Autodesk Fusion 360 part; units mm, degrees
(part 2 of 3)
  line L996 (25.447, -24.192) -> (26.789, -22.378)
  line L997 (26.789, -22.378) -> (26.864, -22.353)
  line L998 (25, -29.138) -> (25.075, -29.163)
  line L999 (25.075, -29.163) -> (26.118, -30.629)
  line L1000 (26.118, -30.629) -> (25.919, -31.026)
  line L1001 (25.919, -31.026) -> (25.025, -32.418)
  line L1002 (25.025, -32.418) -> (24.975, -32.418)
  line L1003 (24.975, -32.418) -> (24.826, -32.219)
  line L1004 (24.826, -32.219) -> (23.907, -30.703)
  line L1005 (23.907, -30.703) -> (23.907, -30.629)
  line L1006 (23.907, -30.629) -> (25, -29.138)
  line L1007 (25, -24.838) -> (25.05, -24.838)
  line L1008 (25.05, -24.838) -> (26.118, -26.354)
  line L1009 (26.118, -26.354) -> (26.118, -26.404)
  line L1010 (26.118, -26.404) -> (25.05, -27.87)
  line L1011 (25.05, -27.87) -> (24.975, -27.87)
  line L1012 (24.975, -27.87) -> (23.907, -26.404)
  line L1013 (23.907, -26.404) -> (23.907, -26.33)
  line L1014 (23.907, -26.33) -> (24.354, -25.683)
  line L1015 (24.354, -25.683) -> (25, -24.838)
  line L1016 (26.491, -27.025) -> (26.566, -27.025)
  line L1017 (26.566, -27.025) -> (26.64, -27.1)
  line L1018 (26.64, -27.1) -> (27.435, -28.268)
  line L1019 (27.435, -28.268) -> (27.435, -28.492)
  line L1020 (27.435, -28.492) -> (26.541, -29.983)
  line L1021 (26.541, -29.983) -> (26.466, -29.958)
  line L1022 (26.466, -29.958) -> (25.447, -28.566)
  line L1023 (25.447, -28.566) -> (25.447, -28.492)
  line L1024 (25.447, -28.492) -> (26.491, -27.025)
  line L1025 (23.459, -27) -> (23.534, -27.025)
  line L1026 (23.534, -27.025) -> (24.578, -28.492)
  line L1027 (24.578, -28.492) -> (24.478, -28.69)
  line L1028 (24.478, -28.69) -> (23.534, -29.983)
  line L1029 (23.534, -29.983) -> (23.484, -29.983)
  line L1030 (23.484, -29.983) -> (23.335, -29.784)
  line L1031 (23.335, -29.784) -> (22.589, -28.516)
  line L1032 (22.589, -28.516) -> (22.614, -28.243)
  line L1033 (22.614, -28.243) -> (23.459, -27)
  line L1034 (20.775, -19.346) -> (20.85, -19.371)
  line L1035 (20.85, -19.371) -> (21.421, -20.042)
  line L1036 (21.421, -20.042) -> (22.714, -21.682)
  line L1037 (22.714, -21.682) -> (22.714, -21.757)
  line L1038 (22.714, -21.757) -> (22.068, -22.975)
  line L1039 (22.068, -22.975) -> (21.993, -22.95)
  line L1040 (21.993, -22.95) -> (21.546, -21.409)
  line L1041 (21.546, -21.409) -> (20.999, -19.943)
  line L1042 (20.999, -19.943) -> (20.75, -19.421)
  line L1043 (20.75, -19.421) -> (20.775, -19.346)
  line L1044 (29.25, -19.346) -> (29.274, -19.421)
  line L1045 (29.274, -19.421) -> (28.951, -20.142)
  line L1046 (28.951, -20.142) -> (28.479, -21.434)
  line L1047 (28.479, -21.434) -> (28.057, -22.9)
  line L1048 (28.057, -22.9) -> (27.957, -22.95)
  line L1049 (27.957, -22.95) -> (27.56, -22.229)
  line L1050 (27.56, -22.229) -> (27.311, -21.682)
  line L1051 (27.311, -21.682) -> (28.28, -20.44)
  line L1052 (28.28, -20.44) -> (29.175, -19.371)
  line L1053 (29.175, -19.371) -> (29.25, -19.346)
  line L1054 (12.972, -15.072) -> (13.519, -15.047)
  line L1055 (13.519, -15.047) -> (13.917, -15.097)
  line L1056 (13.917, -15.097) -> (14.438, -15.221)
  line L1057 (14.438, -15.221) -> (15.383, -15.668)
  line L1058 (15.383, -15.668) -> (15.432, -15.768)
  line L1059 (15.432, -15.768) -> (15.333, -15.818)
  line L1060 (15.333, -15.818) -> (14.96, -15.867)
  line L1061 (14.96, -15.867) -> (14.563, -16.016)
  line L1062 (14.563, -16.016) -> (14.414, -16.016)
  line L1063 (14.414, -16.016) -> (13.593, -15.445)
  line L1064 (13.593, -15.445) -> (12.997, -15.147)
  line L1065 (12.997, -15.147) -> (12.972, -15.072)
  line L1066 (37.053, -15.072) -> (37.003, -15.171)
  line L1067 (37.003, -15.171) -> (36.804, -15.246)
  line L1068 (36.804, -15.246) -> (36.233, -15.569)
  line L1069 (36.233, -15.569) -> (35.611, -16.016)
  line L1070 (35.611, -16.016) -> (35.487, -16.016)
  line L1071 (35.487, -16.016) -> (35.338, -15.942)
  line L1072 (35.338, -15.942) -> (34.841, -15.818)
  line L1073 (34.841, -15.818) -> (34.692, -15.818)
  line L1074 (34.692, -15.818) -> (34.617, -15.768)
  line L1075 (34.617, -15.768) -> (34.667, -15.668)
  line L1076 (34.667, -15.668) -> (34.916, -15.519)
  line L1077 (34.916, -15.519) -> (35.76, -15.171)
  line L1078 (35.76, -15.171) -> (36.506, -15.047)
  line L1079 (36.506, -15.047) -> (37.053, -15.072)
  line L1080 (24.205, -7.517) -> (24.975, -7.12)
  line L1081 (24.975, -7.12) -> (25.075, -7.12)
  line L1082 (25.075, -7.12) -> (25.845, -7.493)
  line L1083 (25.845, -7.493) -> (25.87, -7.567)
  line L1084 (25.87, -7.567) -> (25, -7.99)
  line L1085 (25, -7.99) -> (24.254, -7.617)
  line L1086 (24.254, -7.617) -> (24.205, -7.517)
  line L1087 (27.46, -29.784) -> (27.535, -29.809)
  line L1088 (27.535, -29.809) -> (27.659, -30.877)
  line L1089 (27.659, -30.877) -> (27.808, -31.623)
  line L1090 (27.808, -31.623) -> (27.783, -31.747)
  line L1091 (27.783, -31.747) -> (27.709, -31.722)
  line L1092 (27.709, -31.722) -> (26.963, -30.654)
  line L1093 (26.963, -30.654) -> (26.988, -30.529)
  line L1094 (26.988, -30.529) -> (27.46, -29.784)
  line L1095 (22.565, -29.784) -> (23.037, -30.554)
  line L1096 (23.037, -30.554) -> (23.062, -30.654)
  line L1097 (23.062, -30.654) -> (22.341, -31.672)
  line L1098 (22.341, -31.672) -> (22.266, -31.697)
  line L1099 (22.266, -31.697) -> (22.242, -31.573)
  line L1100 (22.242, -31.573) -> (22.391, -30.753)
  line L1101 (22.391, -30.753) -> (22.49, -29.809)
  line L1102 (22.49, -29.809) -> (22.565, -29.784)
  line L1103 (27.535, -25.634) -> (27.56, -25.808)
  line L1104 (27.56, -25.808) -> (27.46, -26.951)
  line L1105 (27.46, -26.951) -> (27.386, -26.976)
  line L1106 (27.386, -26.976) -> (27.013, -26.479)
  line L1107 (27.013, -26.479) -> (26.988, -26.33)
  line L1108 (26.988, -26.33) -> (27.46, -25.659)
  line L1109 (27.46, -25.659) -> (27.535, -25.634)
  line L1110 (22.49, -25.634) -> (22.565, -25.659)
  line L1111 (22.565, -25.659) -> (23.037, -26.33)
  line L1112 (23.037, -26.33) -> (23.037, -26.429)
  line L1113 (23.037, -26.429) -> (22.639, -26.976)
  line L1114 (22.639, -26.976) -> (22.565, -26.951)
  line L1115 (22.565, -26.951) -> (22.565, -26.553)
  line L1116 (22.565, -26.553) -> (22.465, -25.708)
  line L1117 (22.465, -25.708) -> (22.49, -25.634)
extrude "Extrude1" add sketch "Sketch1" along normal blind 3
sketch "Sketch2" plane through (0, 0, 0) normal (0, 0, 1) x (1, 0, 0)
  circle A0 centre (25, -25) radius 27.5
  circle A1 centre (25, -25) radius 24
  line L0 (24.5, -0.5) -> (25.5, -0.5)
  line L1 (25.5, -0.5) -> (25.5, -6.5)
  line L2 (25.5, -6.5) -> (24.5, -6.5)
  line L3 (24.5, -6.5) -> (24.5, -0.5)
  line L4 (11.009, -44.421) -> (19.21, -44.396)
  line L5 (13.345, -43.725) -> (12.202, -43.7)
  line L6 (37.823, -43.7) -> (36.705, -43.725)
  line L7 (30.691, -44.396) -> (39.041, -44.396)
  line L8 (37.264, -43.7125) -> (40.3407, -43.7125)
  line L9 (40.3407, -43.7125) -> (40.3407, -44.396)
  line L10 (40.3407, -44.396) -> (37.264, -44.396)
  line L11 (37.264, -44.396) -> (37.264, -43.7125)
  line L12 (12.7735, -43.7125) -> (9.7904, -43.7125)
  line L13 (9.7904, -43.7125) -> (9.7904, -44.4085)
  line L14 (9.7904, -44.4085) -> (12.7735, -44.4085)
  line L15 (12.7735, -44.4085) -> (12.7735, -43.7125)
  line L16 (12.351, -11.643) -> (7.306, -13.73)
  line L17 (7.654, -14.476) -> (14.612, -11.593)
  line L18 (42.719, -13.705) -> (39.19, -12.239)
  line L19 (38.917, -13.009) -> (42.371, -14.476)
  line L20 (40.9545, -12.972) -> (40.644, -13.7425)
  line L21 (40.644, -13.7425) -> (47.8102, -16.6302)
  line L22 (47.8102, -16.6302) -> (48.1207, -15.8597)
  line L23 (48.1207, -15.8597) -> (40.9545, -12.972)
  line L24 (9.8285, -12.6865) -> (10.1427, -13.4448)
  line L25 (10.1427, -13.4448) -> (2.127, -16.766)
  line L26 (2.127, -16.766) -> (1.8128, -16.0077)
  line L27 (1.8128, -16.0077) -> (9.8285, -12.6865)
  dimension "d3" = 55
  dimension "d4" = 48
  constraint concentric A0 A1
  constraint horizontal L0
  constraint vertical L1
  constraint horizontal L2
  constraint vertical L3
  constraint horizontal L8
  constraint vertical L9
  constraint horizontal L10
  constraint vertical L11
  constraint midpoint L6 L8.start
  constraint horizontal L12
  constraint vertical L13
  constraint horizontal L14
  constraint vertical L15
  constraint midpoint L5 L12.start
  constraint perpendicular L20 L21
  constraint parallel L20 L22
  constraint parallel L21 L23
  constraint midpoint L19 L20.end
  constraint midpoint L18 L20.start
  constraint perpendicular L24 L25
  constraint parallel L24 L26
  constraint parallel L25 L27
  constraint coincident L17 L24.end
  constraint perpendicular L17 L24
  constraint midpoint L16 L24.start
  measures "d3" diameter of A0
  measures "d4" diameter of A1
extrude "Extrude2" add sketch "Sketch2" along normal blind 3 contours A0 | A1 L20 L21 L23 | A1 L21 L22 L23 | A1 L8 L9 L10 | A1 L7 L8 L10 L11 | A1 L1 L2 L3 | A1 L0 L1 L3 | A1 L12 L13 L14 | A1 L12 L14 L15 | A1 L16 L17 L24 L25 L27 | A1 L25 L26 L27
sketch "Sketch4" plane through (0, 0, 3) normal (0, 0, 1) x (-1, 0, 0)
  arc A0 (-6.803, 9.3517) -> (-2.9434, 15.5393) centre (-25, 25) ccw
  line L0 (-11.1263, 43.7125) -> (-9.9976, 43.7125)
  line L1 (-24.5, 1.0052) -> (-24.5, 5.9525)
  line L2 (-25.5, 5.9758) -> (-25.5, 1.0052)
  line L3 (-40.0281, 43.7125) -> (-38.8766, 43.7125)
  line L4 (-30.691, 44.396) -> (-39.041, 44.396)
  circle A1 centre (-25, 25) radius 27.5
  circle A2 centre (-25, 25) radius 27.5
  circle A3 centre (-25, 25) radius 27.5
  circle A4 centre (-25, 25) radius 25.5
  line L5 (-24.5, 5.9525) -> (-22.639, 4.983)
  line L6 (-22.639, 4.983) -> (-21.993, 4.684)
  line L7 (-21.993, 4.684) -> (-21.645, 5.355)
  line L8 (-21.645, 5.355) -> (-21.695, 5.455)
  line L9 (-21.695, 5.455) -> (-24.006, 6.623)
  line L10 (-24.006, 6.623) -> (-23.981, 6.722)
  line L11 (-23.981, 6.722) -> (-23.236, 7.095)
  line L12 (-23.236, 7.095) -> (-22.913, 6.971)
  line L13 (-22.913, 6.971) -> (-19.135, 5.082)
  line L14 (-19.135, 5.082) -> (-19.036, 5.082)
  line L15 (-19.036, 5.082) -> (-18.738, 5.678)
  line L16 (-18.738, 5.678) -> (-18.713, 5.803)
  line L17 (-18.713, 5.803) -> (-18.762, 5.852)
  line L18 (-18.762, 5.852) -> (-22.142, 7.468)
  line L19 (-22.142, 7.468) -> (-22.167, 7.567)
  line L20 (-22.167, 7.567) -> (-18.588, 9.133)
  line L21 (-18.588, 9.133) -> (-12.351, 11.643)
  line L22 (-12.351, 11.643) -> (-7.306, 13.73)
  line L23 (-7.306, 13.73) -> (-7.3062, 13.7316)
  line L24 (-2.5162, 16.6048) -> (-14.612, 11.593)
  line L25 (-14.612, 11.593) -> (-14.687, 11.593)
  line L26 (-14.687, 11.593) -> (-14.786, 11.692)
  line L27 (-14.786, 11.692) -> (-15.234, 12.338)
  line L28 (-15.234, 12.338) -> (-15.283, 12.363)
  line L29 (-15.283, 12.363) -> (-15.283, 12.413)
  line L30 (-15.283, 12.413) -> (-15.184, 12.488)
  line L31 (-15.184, 12.488) -> (-11.257, 14.327)
  line L32 (-11.257, 14.327) -> (-10.736, 14.401)
  line L33 (-10.736, 14.401) -> (-9.568, 14.476)
  line L34 (-9.568, 14.476) -> (-8.822, 14.6)
  line L35 (-8.822, 14.6) -> (-7.878, 14.873)
  line L36 (-7.878, 14.873) -> (-6.909, 15.321)
  line L37 (-6.909, 15.321) -> (-6.064, 15.867)
  line L38 (-6.064, 15.867) -> (-5.442, 16.389)
  line L39 (-5.442, 16.389) -> (-4.722, 17.16)
  line L40 (-4.722, 17.16) -> (-4.125, 18.004)
  line L41 (-4.125, 18.004) -> (-3.628, 18.949)
  line L42 (-3.628, 18.949) -> (-3.28, 19.794)
  line L43 (-3.28, 19.794) -> (-2.908, 21.061)
  line L44 (-2.908, 21.061) -> (-2.709, 22.229)
  line L45 (-2.709, 22.229) -> (-2.609, 23.397)
  line L46 (-2.609, 23.397) -> (-2.609, 26.18)
  line L47 (-2.609, 26.18) -> (-2.46, 26.255)
  line L48 (-2.46, 26.255) -> (-2.386, 26.379)
  line L49 (-2.386, 26.379) -> (-2.411, 31.772)
  line L50 (-2.411, 31.772) -> (-2.56, 31.871)
  line L51 (-2.56, 31.871) -> (-3.429, 31.846)
  line L52 (-3.429, 31.846) -> (-3.529, 31.747)
  line L53 (-3.529, 31.747) -> (-3.529, 26.354)
  line L54 (-3.529, 26.354) -> (-3.454, 26.255)
  line L55 (-3.454, 26.255) -> (-3.305, 26.18)
  line L56 (-3.305, 26.18) -> (-3.33, 23.298)
  line L57 (-3.33, 23.298) -> (-3.405, 22.403)
  line L58 (-3.405, 22.403) -> (-3.529, 21.608)
  line L59 (-3.529, 21.608) -> (-3.802, 20.539)
  line L60 (-3.802, 20.539) -> (-4.15, 19.57)
  line L61 (-4.15, 19.57) -> (-4.548, 18.75)
  line L62 (-4.548, 18.75) -> (-5.119, 17.855)
  line L63 (-5.119, 17.855) -> (-5.567, 17.309)
  line L64 (-5.567, 17.309) -> (-6.362, 16.563)
  line L65 (-6.362, 16.563) -> (-7.083, 16.066)
  line L66 (-7.083, 16.066) -> (-7.853, 15.668)
  line L67 (-7.853, 15.668) -> (-8.549, 15.42)
  line L68 (-8.549, 15.42) -> (-9.493, 15.221)
  line L69 (-9.493, 15.221) -> (-10.437, 15.196)
  line L70 (-10.437, 15.196) -> (-10.487, 15.296)
  line L71 (-10.487, 15.296) -> (-9.965, 15.619)
  line L72 (-9.965, 15.619) -> (-9.195, 16.215)
  line L73 (-9.195, 16.215) -> (-8.499, 16.911)
  line L74 (-8.499, 16.911) -> (-7.977, 17.582)
  line L75 (-7.977, 17.582) -> (-7.455, 18.427)
  line L76 (-7.455, 18.427) -> (-7.083, 19.197)
  line L77 (-7.083, 19.197) -> (-6.759, 20.067)
  line L78 (-6.759, 20.067) -> (-6.436, 21.334)
  line L79 (-6.436, 21.334) -> (-6.312, 22.105)
  line L80 (-6.312, 22.105) -> (-6.213, 23.173)
  line L81 (-6.213, 23.173) -> (-6.213, 28.019)
  line L82 (-6.213, 28.019) -> (-6.188, 28.119)
  line L83 (-6.188, 28.119) -> (-6.039, 28.268)
  line L84 (-6.039, 28.268) -> (-6.039, 34.307)
  line L85 (-6.039, 34.307) -> (-6.163, 34.406)
  line L86 (-6.163, 34.406) -> (-7.058, 34.406)
  line L87 (-7.058, 34.406) -> (-7.182, 34.282)
  line L88 (-7.182, 34.282) -> (-7.182, 28.268)
  line L89 (-7.182, 28.268) -> (-7.058, 28.144)
  line L90 (-7.058, 28.144) -> (-6.958, 28.144)
  line L91 (-6.958, 28.144) -> (-6.909, 28.094)
  line L92 (-6.909, 28.094) -> (-6.909, 23.571)
  line L93 (-6.909, 23.571) -> (-6.983, 22.478)
  line L94 (-6.983, 22.478) -> (-7.058, 21.956)
  line L95 (-7.058, 21.956) -> (-7.381, 20.514)
  line L96 (-7.381, 20.514) -> (-7.629, 19.794)
  line L97 (-7.629, 19.794) -> (-8.077, 18.825)
  line L98 (-8.077, 18.825) -> (-8.499, 18.129)
  line L99 (-8.499, 18.129) -> (-9.046, 17.408)
  line L100 (-9.046, 17.408) -> (-9.717, 16.737)
  line L101 (-9.717, 16.737) -> (-10.288, 16.29)
  line L102 (-10.288, 16.29) -> (-11.108, 15.793)
  line L103 (-11.108, 15.793) -> (-11.655, 15.544)
  line L104 (-11.655, 15.544) -> (-11.953, 15.495)
  line L105 (-11.953, 15.495) -> (-12.525, 15.718)
  line L106 (-12.525, 15.718) -> (-13.37, 16.166)
  line L107 (-13.37, 16.166) -> (-13.593, 16.315)
  line L108 (-13.593, 16.315) -> (-13.643, 16.414)
  line L109 (-13.643, 16.414) -> (-13.121, 16.787)
  line L110 (-13.121, 16.787) -> (-12.724, 17.16)
  line L111 (-12.724, 17.16) -> (-12.401, 17.532)
  line L112 (-12.401, 17.532) -> (-11.978, 18.154)
  line L113 (-11.978, 18.154) -> (-11.754, 18.551)
  line L114 (-11.754, 18.551) -> (-11.307, 19.595)
  line L115 (-11.307, 19.595) -> (-11.059, 20.415)
  line L116 (-11.059, 20.415) -> (-10.91, 21.061)
  line L117 (-10.91, 21.061) -> (-10.785, 21.807)
  line L118 (-10.785, 21.807) -> (-10.661, 23.248)
  line L119 (-10.661, 23.248) -> (-10.686, 26.379)
  line L120 (-10.686, 26.379) -> (-10.661, 26.653)
  line L121 (-10.661, 26.653) -> (-10.562, 26.702)
  line L122 (-10.562, 26.702) -> (-10.462, 26.827)
  line L123 (-10.462, 26.827) -> (-10.487, 33.064)
  line L124 (-10.487, 33.064) -> (-10.586, 33.139)
  line L125 (-10.586, 33.139) -> (-11.506, 33.139)
  line L126 (-11.506, 33.139) -> (-11.605, 33.064)
  line L127 (-11.605, 33.064) -> (-11.63, 32.99)
  line L128 (-11.63, 32.99) -> (-11.63, 26.827)
  line L129 (-11.63, 26.827) -> (-11.531, 26.702)
  line L130 (-11.531, 26.702) -> (-11.407, 26.677)
  line L131 (-11.407, 26.677) -> (-11.357, 26.628)
  line L132 (-11.357, 26.628) -> (-11.357, 23.646)
  line L133 (-11.357, 23.646) -> (-11.481, 22.03)
  line L134 (-11.481, 22.03) -> (-11.655, 21.036)
  line L135 (-11.655, 21.036) -> (-12.003, 19.794)
  line L136 (-12.003, 19.794) -> (-12.251, 19.197)
  line L137 (-12.251, 19.197) -> (-12.649, 18.452)
  line L138 (-12.649, 18.452) -> (-13.022, 17.93)
  line L139 (-13.022, 17.93) -> (-13.469, 17.458)
  line L140 (-13.469, 17.458) -> (-13.743, 17.234)
  line L141 (-13.743, 17.234) -> (-14.314, 16.886)
  line L142 (-14.314, 16.886) -> (-14.364, 16.886)
  line L143 (-14.364, 16.886) -> (-15.283, 17.806)
  line L144 (-15.283, 17.806) -> (-15.656, 18.253)
  line L145 (-15.656, 18.253) -> (-16.352, 19.222)
  line L146 (-16.352, 19.222) -> (-16.923, 20.167)
  line L147 (-16.923, 20.167) -> (-17.321, 20.937)
  line L148 (-17.321, 20.937) -> (-18.017, 22.577)
  line L149 (-18.017, 22.577) -> (-18.489, 24.043)
  line L150 (-18.489, 24.043) -> (-18.688, 24.838)
  line L151 (-18.688, 24.838) -> (-18.887, 25.932)
  line L152 (-18.887, 25.932) -> (-19.036, 27.547)
  line L153 (-19.036, 27.547) -> (-19.011, 29.386)
  line L154 (-19.011, 29.386) -> (-18.812, 30.877)
  line L155 (-18.812, 30.877) -> (-18.415, 32.468)
  line L156 (-18.415, 32.468) -> (-18.216, 33.064)
  line L157 (-18.216, 33.064) -> (-17.52, 34.704)
  line L158 (-17.52, 34.704) -> (-16.874, 35.922)
  line L159 (-16.874, 35.922) -> (-15.979, 37.413)
  line L160 (-15.979, 37.413) -> (-14.314, 39.824)
  line L161 (-14.314, 39.824) -> (-12.798, 41.762)
  line L162 (-12.798, 41.762) -> (-11.1263, 43.7125)
  line L163 (-9.9976, 43.7125) -> (-9.568, 43.377)
  line L164 (-9.568, 43.377) -> (-8.8988, 42.7975)
  line L165 (-8.7235, 42.6374) -> (-8.2028, 42.1422)
  arc A5 (-2.5162, 16.6048) -> (-8.2028, 42.1422) centre (-25, 25) ccw
  line L166 (-6.803, 9.3517) -> (-6.9294, 9.2059)
  arc A6 (-7.6077, 8.4619) -> (-6.9294, 9.2059) centre (-25, 25) ccw
  line L167 (-7.6077, 8.4619) -> (-8.7441, 7.3437)
  arc A7 (-24.5, 1.0052) -> (-8.7441, 7.3437) centre (-25, 25) ccw
  line L168 (-37.823, 43.7) -> (-36.705, 43.725)
  line L169 (-36.705, 43.725) -> (-36.605, 43.675)
  line L170 (-36.605, 43.675) -> (-34.742, 41.315)
  line L171 (-34.742, 41.315) -> (-33.772, 39.948)
  line L172 (-33.772, 39.948) -> (-32.753, 38.382)
  line L173 (-32.753, 38.382) -> (-32.107, 37.264)
  line L174 (-32.107, 37.264) -> (-31.561, 36.195)
  line L175 (-31.561, 36.195) -> (-30.865, 34.555)
  line L176 (-30.865, 34.555) -> (-30.467, 33.412)
  line L177 (-30.467, 33.412) -> (-30.219, 32.542)
  line L178 (-30.219, 32.542) -> (-29.995, 31.598)
  line L179 (-29.995, 31.598) -> (-29.821, 30.629)
  line L180 (-29.821, 30.629) -> (-29.647, 29.138)
  line L181 (-29.647, 29.138) -> (-29.622, 27.274)
  line L182 (-29.622, 27.274) -> (-29.821, 25.261)
  line L183 (-29.821, 25.261) -> (-30.244, 23.298)
  line L184 (-30.244, 23.298) -> (-30.517, 22.378)
  line L185 (-30.517, 22.378) -> (-30.989, 21.061)
  line L186 (-30.989, 21.061) -> (-31.809, 19.247)
  line L187 (-31.809, 19.247) -> (-32.306, 18.352)
  line L188 (-32.306, 18.352) -> (-32.828, 17.532)
  line L189 (-32.828, 17.532) -> (-33.648, 16.513)
  line L190 (-33.648, 16.513) -> (-34.468, 16.513)
  line L191 (-34.468, 16.513) -> (-34.816, 16.588)
  line L192 (-34.816, 16.588) -> (-34.841, 16.663)
  line L193 (-34.841, 16.663) -> (-34.319, 17.184)
  line L194 (-34.319, 17.184) -> (-33.623, 18.029)
  line L195 (-33.623, 18.029) -> (-33.101, 18.775)
  line L196 (-33.101, 18.775) -> (-32.455, 19.843)
  line L197 (-32.455, 19.843) -> (-31.635, 21.558)
  line L198 (-31.635, 21.558) -> (-30.989, 23.372)
  line L199 (-30.989, 23.372) -> (-30.741, 24.292)
  line L200 (-30.741, 24.292) -> (-30.542, 25.236)
  line L201 (-30.542, 25.236) -> (-30.293, 27.174)
  line L202 (-30.293, 27.174) -> (-30.268, 28.765)
  line L203 (-30.268, 28.765) -> (-30.417, 30.38)
  line L204 (-30.417, 30.38) -> (-30.741, 31.971)
  line L205 (-30.741, 31.971) -> (-31.188, 33.412)
  line L206 (-31.188, 33.412) -> (-31.71, 34.679)
  line L207 (-31.71, 34.679) -> (-32.455, 36.146)
  line L208 (-32.455, 36.146) -> (-33.499, 37.885)
  line L209 (-33.499, 37.885) -> (-34.766, 39.749)
  line L210 (-34.766, 39.749) -> (-36.357, 41.861)
  line L211 (-36.357, 41.861) -> (-37.848, 43.626)
  line L212 (-37.848, 43.626) -> (-37.823, 43.7)
  line L213 (-21.421, 34.878) -> (-21.595, 34.232)
  line L214 (-21.595, 34.232) -> (-21.67, 34.207)
  line L215 (-21.67, 34.207) -> (-21.769, 34.406)
  line L216 (-21.769, 34.406) -> (-22.291, 35.997)
  line L217 (-22.291, 35.997) -> (-22.465, 36.419)
  line L218 (-22.465, 36.419) -> (-22.515, 36.667)
  line L219 (-22.515, 36.667) -> (-20.8, 39.55)
  line L220 (-20.8, 39.55) -> (-19.98, 41.016)
  line L221 (-19.98, 41.016) -> (-19.185, 42.607)
  line L222 (-19.185, 42.607) -> (-18.762, 43.675)
  line L223 (-18.762, 43.675) -> (-18.688, 43.725)
  line L224 (-18.688, 43.725) -> (-17.768, 43.725)
  line L225 (-17.768, 43.725) -> (-17.719, 43.675)
  line L226 (-17.719, 43.675) -> (-17.744, 43.551)
  line L227 (-17.744, 43.551) -> (-18.986, 41.016)
  line L228 (-18.986, 41.016) -> (-20.179, 38.258)
  line L229 (-20.179, 38.258) -> (-20.949, 36.27)
  line L230 (-20.949, 36.27) -> (-21.421, 34.878)
  line L231 (-30.915, 17.756) -> (-31.436, 16.911)
  line L232 (-31.436, 16.911) -> (-31.735, 16.513)
  line L233 (-31.735, 16.513) -> (-32.604, 16.513)
  line L234 (-32.604, 16.513) -> (-32.629, 16.588)
  line L235 (-32.629, 16.588) -> (-32.281, 17.035)
  line L236 (-32.281, 17.035) -> (-31.561, 18.178)
  line L237 (-31.561, 18.178) -> (-30.815, 19.62)
  line L238 (-30.815, 19.62) -> (-30.442, 20.465)
  line L239 (-30.442, 20.465) -> (-30.094, 21.359)
  line L240 (-30.094, 21.359) -> (-29.722, 22.478)
  line L241 (-29.722, 22.478) -> (-29.25, 24.366)
  line L242 (-29.25, 24.366) -> (-29.001, 25.957)
  line L243 (-29.001, 25.957) -> (-28.902, 27.398)
  line L244 (-28.902, 27.398) -> (-28.926, 29.138)
  line L245 (-28.926, 29.138) -> (-29.051, 30.331)
  line L246 (-29.051, 30.331) -> (-29.349, 31.971)
  line L247 (-29.349, 31.971) -> (-29.771, 33.586)
  line L248 (-29.771, 33.586) -> (-29.97, 34.207)
  line L249 (-29.97, 34.207) -> (-30.492, 35.549)
  line L250 (-30.492, 35.549) -> (-31.064, 36.792)
  line L251 (-31.064, 36.792) -> (-31.759, 38.109)
  line L252 (-31.759, 38.109) -> (-32.654, 39.575)
  line L253 (-32.654, 39.575) -> (-33.971, 41.489)
  line L254 (-33.971, 41.489) -> (-35.487, 43.452)
  line L255 (-35.487, 43.452) -> (-35.661, 43.626)
  line L256 (-35.661, 43.626) -> (-35.636, 43.725)
  line L257 (-35.636, 43.725) -> (-33.077, 43.725)
  line L258 (-33.077, 43.725) -> (-33.002, 43.675)
  line L259 (-33.002, 43.675) -> (-31.809, 41.091)
  line L260 (-31.809, 41.091) -> (-31.784, 40.967)
  line L261 (-31.784, 40.967) -> (-31.735, 40.917)
  line L262 (-31.735, 40.917) -> (-30.268, 37.363)
  line L263 (-30.268, 37.363) -> (-29.573, 35.475)
  line L264 (-29.573, 35.475) -> (-28.926, 33.412)
  line L265 (-28.926, 33.412) -> (-28.628, 32.169)
  line L266 (-28.628, 32.169) -> (-28.33, 30.554)
  line L267 (-28.33, 30.554) -> (-28.181, 29.138)
  line L268 (-28.181, 29.138) -> (-28.156, 27.224)
  line L269 (-28.156, 27.224) -> (-28.33, 25.186)
  line L270 (-28.33, 25.186) -> (-28.653, 23.472)
  line L271 (-28.653, 23.472) -> (-28.951, 22.329)
  line L272 (-28.951, 22.329) -> (-29.25, 21.434)
  line L273 (-29.25, 21.434) -> (-29.92, 19.719)
  line L274 (-29.92, 19.719) -> (-30.517, 18.477)
  line L275 (-30.517, 18.477) -> (-30.915, 17.756)
  line L276 (-22.465, 10.077) -> (-23.111, 9.829)
  line L277 (-23.111, 9.829) -> (-24.975, 8.909)
  line L278 (-24.975, 8.909) -> (-25.075, 8.909)
  line L279 (-25.075, 8.909) -> (-26.789, 9.754)
  line L280 (-26.789, 9.754) -> (-27.584, 10.077)
  line L281 (-27.584, 10.077) -> (-27.709, 10.226)
  line L282 (-27.709, 10.226) -> (-28.355, 11.295)
  line L283 (-28.355, 11.295) -> (-28.305, 11.469)
  line L284 (-28.305, 11.469) -> (-26.69, 14.202)
  line L285 (-26.69, 14.202) -> (-25.919, 15.594)
  line L286 (-25.919, 15.594) -> (-25.845, 15.668)
  line L287 (-25.845, 15.668) -> (-25.447, 15.668)
  line L288 (-25.447, 15.668) -> (-25.398, 15.619)
  line L289 (-25.398, 15.619) -> (-25.398, 13.879)
  line L290 (-25.398, 13.879) -> (-25.348, 13.854)
  line L291 (-25.348, 13.854) -> (-24.677, 13.854)
  line L292 (-24.677, 13.854) -> (-24.627, 13.904)
  line L293 (-24.627, 13.904) -> (-24.627, 15.619)
  line L294 (-24.627, 15.619) -> (-24.578, 15.668)
  line L295 (-24.578, 15.668) -> (-24.205, 15.668)
  line L296 (-24.205, 15.668) -> (-24.105, 15.569)
  line L297 (-24.105, 15.569) -> (-21.67, 11.369)
  line L298 (-21.67, 11.369) -> (-21.67, 11.295)
  line L299 (-21.67, 11.295) -> (-22.266, 10.326)
  line L300 (-22.266, 10.326) -> (-22.465, 10.077)
  line L301 (-34.195, 13.109) -> (-34.418, 13.159)
  line L302 (-34.418, 13.159) -> (-36.73, 14.252)
  line L303 (-36.73, 14.252) -> (-36.705, 14.327)
  line L304 (-36.705, 14.327) -> (-36.108, 14.351)
  line L305 (-36.108, 14.351) -> (-35.537, 14.476)
  line L306 (-35.537, 14.476) -> (-34.866, 14.724)
  line L307 (-34.866, 14.724) -> (-34.195, 15.097)
  line L308 (-34.195, 15.097) -> (-33.474, 15.668)
  line L309 (-33.474, 15.668) -> (-32.406, 15.644)
  line L310 (-32.406, 15.644) -> (-32.43, 15.544)
  line L311 (-32.43, 15.544) -> (-34.195, 13.109)
  line L312 (-18.216, 11.941) -> (-21.098, 10.649)
  line L313 (-21.098, 10.649) -> (-21.173, 10.649)
  line L314 (-21.173, 10.649) -> (-21.198, 10.748)
  line L315 (-21.198, 10.748) -> (-18.588, 15.072)
  line L316 (-18.588, 15.072) -> (-18.464, 15.271)
  line L317 (-18.464, 15.271) -> (-18.365, 15.321)
  line L318 (-18.365, 15.321) -> (-16.526, 12.811)
  line L319 (-16.526, 12.811) -> (-16.526, 12.761)
  line L320 (-16.526, 12.761) -> (-16.998, 12.512)
  line L321 (-16.998, 12.512) -> (-18.017, 12.065)
  line L322 (-18.017, 12.065) -> (-18.216, 11.941)
  line L323 (-13.693, 14.327) -> (-13.345, 14.327)
  line L324 (-13.345, 14.327) -> (-13.32, 14.252)
  line L325 (-13.32, 14.252) -> (-15.731, 13.109)
  line L326 (-15.731, 13.109) -> (-15.83, 13.109)
  line L327 (-15.83, 13.109) -> (-17.644, 15.594)
  line L328 (-17.644, 15.594) -> (-17.644, 15.644)
  line L329 (-17.644, 15.644) -> (-16.551, 15.668)
  line L330 (-16.551, 15.668) -> (-16.153, 15.321)
  line L331 (-16.153, 15.321) -> (-15.606, 14.948)
  line L332 (-15.606, 14.948) -> (-15.01, 14.65)
  line L333 (-15.01, 14.65) -> (-14.314, 14.426)
  line L334 (-14.314, 14.426) -> (-13.693, 14.327)
  line L335 (-23.907, 30.703) -> (-23.907, 30.629)
  line L336 (-23.907, 30.629) -> (-25, 29.138)
  line L337 (-25, 29.138) -> (-25.075, 29.163)
  line L338 (-25.075, 29.163) -> (-26.118, 30.629)
  line L339 (-26.118, 30.629) -> (-25.919, 31.026)
  line L340 (-25.919, 31.026) -> (-25.025, 32.418)
  line L341 (-25.025, 32.418) -> (-24.975, 32.418)
  line L342 (-24.975, 32.418) -> (-24.826, 32.219)
  line L343 (-24.826, 32.219) -> (-23.907, 30.703)
  line L344 (-26.963, 30.654) -> (-26.988, 30.529)
  line L345 (-26.988, 30.529) -> (-27.46, 29.784)
  line L346 (-27.46, 29.784) -> (-27.535, 29.809)
  line L347 (-27.535, 29.809) -> (-27.659, 30.877)
  line L348 (-27.659, 30.877) -> (-27.808, 31.623)
  line L349 (-27.808, 31.623) -> (-27.783, 31.747)
  line L350 (-27.783, 31.747) -> (-27.709, 31.722)
  line L351 (-27.709, 31.722) -> (-26.963, 30.654)
  line L352 (-25, 7.99) -> (-24.254, 7.617)
  line L353 (-24.254, 7.617) -> (-24.205, 7.517)
  line L354 (-24.205, 7.517) -> (-24.975, 7.12)
  line L355 (-24.975, 7.12) -> (-25.075, 7.12)
  line L356 (-25.075, 7.12) -> (-25.845, 7.493)
  line L357 (-25.845, 7.493) -> (-25.87, 7.567)
  line L358 (-25.87, 7.567) -> (-25, 7.99)
  line L359 (-29.15, 11.245) -> (-28.802, 10.698)
  line L360 (-28.802, 10.698) -> (-28.827, 10.624)
  line L361 (-28.827, 10.624) -> (-30.144, 11.17)
  line L362 (-30.144, 11.17) -> (-33.499, 12.736)
  line L363 (-33.499, 12.736) -> (-33.499, 12.811)
  line L364 (-33.499, 12.811) -> (-32.207, 14.55)
  line L365 (-32.207, 14.55) -> (-31.66, 15.345)
  line L366 (-31.66, 15.345) -> (-31.561, 15.296)
  line L367 (-31.561, 15.296) -> (-31.412, 14.998)
  line L368 (-31.412, 14.998) -> (-29.97, 12.662)
  line L369 (-29.97, 12.662) -> (-29.15, 11.245)
  line L370 (-28.28, 20.44) -> (-29.175, 19.371)
  line L371 (-29.175, 19.371) -> (-29.25, 19.346)
  line L372 (-29.25, 19.346) -> (-29.274, 19.421)
  line L373 (-29.274, 19.421) -> (-28.951, 20.142)
  line L374 (-28.951, 20.142) -> (-28.479, 21.434)
  line L375 (-28.479, 21.434) -> (-28.057, 22.9)
  line L376 (-28.057, 22.9) -> (-27.957, 22.95)
  line L377 (-27.957, 22.95) -> (-27.56, 22.229)
  line L378 (-27.56, 22.229) -> (-27.311, 21.682)
  line L379 (-27.311, 21.682) -> (-28.28, 20.44)
  line L380 (-21.297, 18.825) -> (-19.284, 16.588)
  line L381 (-19.284, 16.588) -> (-19.309, 16.513)
  line L382 (-19.309, 16.513) -> (-23.882, 16.513)
  line L383 (-23.882, 16.513) -> (-23.956, 16.588)
  line L384 (-23.956, 16.588) -> (-24.553, 17.607)
  line L385 (-24.553, 17.607) -> (-24.627, 17.831)
  line L386 (-24.627, 17.831) -> (-23.683, 19.843)
  line L387 (-23.683, 19.843) -> (-23.086, 20.987)
  line L388 (-23.086, 20.987) -> (-23.012, 20.962)
  line L389 (-23.012, 20.962) -> (-21.297, 18.825)
  line L390 (-22.391, 30.753) -> (-22.49, 29.809)
  line L391 (-22.49, 29.809) -> (-22.565, 29.784)
  line L392 (-22.565, 29.784) -> (-23.037, 30.554)
  line L393 (-23.037, 30.554) -> (-23.062, 30.654)
  line L394 (-23.062, 30.654) -> (-22.341, 31.672)
  line L395 (-22.341, 31.672) -> (-22.266, 31.697)
  line L396 (-22.266, 31.697) -> (-22.242, 31.573)
  line L397 (-22.242, 31.573) -> (-22.391, 30.753)
  line L398 (-22.266, 24.118) -> (-22.316, 23.944)
  line L399 (-22.316, 23.944) -> (-23.161, 22.378)
  line L400 (-23.161, 22.378) -> (-23.236, 22.378)
  line L401 (-23.236, 22.378) -> (-24.578, 24.167)
  line L402 (-24.578, 24.167) -> (-24.578, 24.267)
  line L403 (-24.578, 24.267) -> (-23.509, 25.733)
  line L404 (-23.509, 25.733) -> (-23.41, 25.708)
  line L405 (-23.41, 25.708) -> (-22.266, 24.118)
  line L406 (-26.988, 26.33) -> (-27.46, 25.659)
  line L407 (-27.46, 25.659) -> (-27.535, 25.634)
  line L408 (-27.535, 25.634) -> (-27.56, 25.808)
  line L409 (-27.56, 25.808) -> (-27.46, 26.951)
  line L410 (-27.46, 26.951) -> (-27.386, 26.976)
  line L411 (-27.386, 26.976) -> (-27.013, 26.479)
  line L412 (-27.013, 26.479) -> (-26.988, 26.33)
  line L413 (-20.999, 19.943) -> (-20.75, 19.421)
  line L414 (-20.75, 19.421) -> (-20.775, 19.346)
  line L415 (-20.775, 19.346) -> (-20.85, 19.371)
  line L416 (-20.85, 19.371) -> (-21.421, 20.042)
  line L417 (-21.421, 20.042) -> (-22.714, 21.682)
  line L418 (-22.714, 21.682) -> (-22.714, 21.757)
  line L419 (-22.714, 21.757) -> (-22.068, 22.975)
  line L420 (-22.068, 22.975) -> (-21.993, 22.95)
  line L421 (-21.993, 22.95) -> (-21.546, 21.409)
  line L422 (-21.546, 21.409) -> (-20.999, 19.943)
  line L423 (-30.964, 15.644) -> (-26.715, 15.668)
  line L424 (-26.715, 15.668) -> (-26.69, 15.594)
  line L425 (-26.69, 15.594) -> (-28.752, 12.065)
  line L426 (-28.752, 12.065) -> (-28.827, 12.065)
  line L427 (-28.827, 12.065) -> (-30.741, 15.196)
  line L428 (-30.741, 15.196) -> (-30.964, 15.644)
  line L429 (-27.063, 8.959) -> (-26.069, 8.487)
  line L430 (-26.069, 8.487) -> (-26.044, 8.412)
  line L431 (-26.044, 8.412) -> (-26.74, 8.039)
  line L432 (-26.74, 8.039) -> (-26.914, 7.99)
  line L433 (-26.914, 7.99) -> (-27.982, 8.487)
  line L434 (-27.982, 8.487) -> (-29.1, 8.934)
  line L435 (-29.1, 8.934) -> (-30.666, 9.63)
  line L436 (-30.666, 9.63) -> (-34.617, 11.245)
  line L437 (-34.617, 11.245) -> (-34.642, 11.32)
  line L438 (-34.642, 11.32) -> (-34.071, 12.065)
  line L439 (-34.071, 12.065) -> (-33.971, 12.065)
  line L440 (-33.971, 12.065) -> (-31.362, 10.823)
  line L441 (-31.362, 10.823) -> (-27.063, 8.959)
  line L442 (-25.447, 28.566) -> (-25.447, 28.492)
  line L443 (-25.447, 28.492) -> (-26.491, 27.025)
  line L444 (-26.491, 27.025) -> (-26.566, 27.025)
  line L445 (-26.566, 27.025) -> (-26.64, 27.1)
  line L446 (-26.64, 27.1) -> (-27.435, 28.268)
  line L447 (-27.435, 28.268) -> (-27.435, 28.492)
  line L448 (-27.435, 28.492) -> (-26.541, 29.983)
  line L449 (-26.541, 29.983) -> (-26.466, 29.958)
  line L450 (-26.466, 29.958) -> (-25.447, 28.566)
  line L451 (-23.559, 21.658) -> (-23.559, 21.583)
  line L452 (-23.559, 21.583) -> (-25, 18.651)
  line L453 (-25, 18.651) -> (-25.05, 18.651)
  line L454 (-25.05, 18.651) -> (-25.149, 18.8)
  line L455 (-25.149, 18.8) -> (-26.168, 20.987)
  line L456 (-26.168, 20.987) -> (-26.491, 21.583)
  line L457 (-26.491, 21.583) -> (-26.491, 21.682)
  line L458 (-26.491, 21.682) -> (-25.05, 23.596)
  line L459 (-25.05, 23.596) -> (-25, 23.596)
  line L460 (-25, 23.596) -> (-24.876, 23.472)
  line L461 (-24.876, 23.472) -> (-23.559, 21.658)
  line L462 (-35.76, 15.171) -> (-36.506, 15.047)
  line L463 (-36.506, 15.047) -> (-37.053, 15.072)
  line L464 (-37.053, 15.072) -> (-37.003, 15.171)
  line L465 (-37.003, 15.171) -> (-36.804, 15.246)
  line L466 (-36.804, 15.246) -> (-36.233, 15.569)
  line L467 (-36.233, 15.569) -> (-35.611, 16.016)
  line L468 (-35.611, 16.016) -> (-35.487, 16.016)
  line L469 (-35.487, 16.016) -> (-35.338, 15.942)
  line L470 (-35.338, 15.942) -> (-34.841, 15.818)
  line L471 (-34.841, 15.818) -> (-34.692, 15.818)
  line L472 (-34.692, 15.818) -> (-34.617, 15.768)
  line L473 (-34.617, 15.768) -> (-34.667, 15.668)
  line L474 (-34.667, 15.668) -> (-34.916, 15.519)
  line L475 (-34.916, 15.519) -> (-35.76, 15.171)
  line L476 (-13.593, 15.445) -> (-12.997, 15.147)
  line L477 (-12.997, 15.147) -> (-12.972, 15.072)
  line L478 (-12.972, 15.072) -> (-13.519, 15.047)
  line L479 (-13.519, 15.047) -> (-13.917, 15.097)
  line L480 (-13.917, 15.097) -> (-14.438, 15.221)
  line L481 (-14.438, 15.221) -> (-15.383, 15.668)
  line L482 (-15.383, 15.668) -> (-15.432, 15.768)
  line L483 (-15.432, 15.768) -> (-15.333, 15.818)
  line L484 (-15.333, 15.818) -> (-14.96, 15.867)
  line L485 (-14.96, 15.867) -> (-14.563, 16.016)
  line L486 (-14.563, 16.016) -> (-14.414, 16.016)
  line L487 (-14.414, 16.016) -> (-13.593, 15.445)
  line L488 (-25.447, 24.192) -> (-26.789, 22.378)
  line L489 (-26.789, 22.378) -> (-26.864, 22.353)
  line L490 (-26.864, 22.353) -> (-27.758, 24.093)
  line L491 (-27.758, 24.093) -> (-26.566, 25.733)
  line L492 (-26.566, 25.733) -> (-26.516, 25.733)
  line L493 (-26.516, 25.733) -> (-25.497, 24.317)
  line L494 (-25.497, 24.317) -> (-25.447, 24.192)
  line L495 (-22.565, 26.553) -> (-22.465, 25.708)
  line L496 (-22.465, 25.708) -> (-22.49, 25.634)
  line L497 (-22.49, 25.634) -> (-22.565, 25.659)
  line L498 (-22.565, 25.659) -> (-23.037, 26.33)
  line L499 (-23.037, 26.33) -> (-23.037, 26.429)
  line L500 (-23.037, 26.429) -> (-22.639, 26.976)
  line L501 (-22.639, 26.976) -> (-22.565, 26.951)
  line L502 (-22.565, 26.951) -> (-22.565, 26.553)
  line L503 (-22.589, 28.516) -> (-22.614, 28.243)
  line L504 (-22.614, 28.243) -> (-23.459, 27)
  line L505 (-23.459, 27) -> (-23.534, 27.025)
  line L506 (-23.534, 27.025) -> (-24.578, 28.492)
  line L507 (-24.578, 28.492) -> (-24.478, 28.69)
  line L508 (-24.478, 28.69) -> (-23.534, 29.983)
  line L509 (-23.534, 29.983) -> (-23.484, 29.983)
  line L510 (-23.484, 29.983) -> (-23.335, 29.784)
  line L511 (-23.335, 29.784) -> (-22.589, 28.516)
  line L512 (-23.062, 8.039) -> (-23.285, 8.039)
  line L513 (-23.285, 8.039) -> (-24.006, 8.412)
  line L514 (-24.006, 8.412) -> (-23.981, 8.487)
  line L515 (-23.981, 8.487) -> (-22.639, 9.133)
  line L516 (-22.639, 9.133) -> (-19.583, 10.425)
  line L517 (-19.583, 10.425) -> (-19.483, 10.5)
  line L518 (-19.483, 10.5) -> (-16.923, 11.643)
  line L519 (-16.923, 11.643) -> (-16.029, 12.09)
  line L520 (-16.029, 12.09) -> (-15.954, 12.065)
  line L521 (-15.954, 12.065) -> (-15.408, 11.344)
  line L522 (-15.408, 11.344) -> (-15.408, 11.295)
  line L523 (-15.408, 11.295) -> (-15.507, 11.22)
  line L524 (-15.507, 11.22) -> (-19.93, 9.431)
  line L525 (-19.93, 9.431) -> (-20.154, 9.307)
  line L526 (-20.154, 9.307) -> (-22.565, 8.288)
  line L527 (-22.565, 8.288) -> (-23.062, 8.039)
  line L528 (-23.907, 26.33) -> (-24.354, 25.683)
  line L529 (-24.354, 25.683) -> (-25, 24.838)
  line L530 (-25, 24.838) -> (-25.05, 24.838)
  line L531 (-25.05, 24.838) -> (-26.118, 26.354)
  line L532 (-26.118, 26.354) -> (-26.118, 26.404)
  line L533 (-26.118, 26.404) -> (-25.05, 27.87)
  line L534 (-25.05, 27.87) -> (-24.975, 27.87)
  line L535 (-24.975, 27.87) -> (-23.907, 26.404)
  line L536 (-23.907, 26.404) -> (-23.907, 26.33)
  line L537 (-23.36, 15.644) -> (-19.085, 15.668)
  line L538 (-19.085, 15.668) -> (-19.061, 15.594)
  line L539 (-19.061, 15.594) -> (-21.173, 12.09)
  line L540 (-21.173, 12.09) -> (-21.272, 12.065)
  line L541 (-21.272, 12.065) -> (-22.639, 14.351)
  line L542 (-22.639, 14.351) -> (-23.36, 15.644)
  line L543 (-25.398, 33.164) -> (-25.77, 32.493)
  line L544 (-25.77, 32.493) -> (-26.541, 31.3)
  line L545 (-26.541, 31.3) -> (-26.59, 31.3)
  line L546 (-26.59, 31.3) -> (-27.932, 33.188)
  line L547 (-27.932, 33.188) -> (-27.932, 33.313)
  line L548 (-27.932, 33.313) -> (-27.112, 35.698)
  line L549 (-27.112, 35.698) -> (-27.038, 35.823)
  line L550 (-27.038, 35.823) -> (-26.963, 35.798)
  line L551 (-26.963, 35.798) -> (-26.093, 34.282)
  line L552 (-26.093, 34.282) -> (-25.398, 33.164)
  line L553 (-22.068, 33.188) -> (-23.41, 31.325)
  line L554 (-23.41, 31.325) -> (-23.484, 31.3)
  line L555 (-23.484, 31.3) -> (-24.578, 33.064)
  line L556 (-24.578, 33.064) -> (-24.602, 33.164)
  line L557 (-24.602, 33.164) -> (-23.559, 34.853)
  line L558 (-23.559, 34.853) -> (-23.037, 35.773)
  line L559 (-23.037, 35.773) -> (-22.937, 35.798)
  line L560 (-22.937, 35.798) -> (-22.639, 35.002)
  line L561 (-22.639, 35.002) -> (-22.44, 34.332)
  line L562 (-22.44, 34.332) -> (-22.316, 34.058)
  line L563 (-22.316, 34.058) -> (-22.068, 33.313)
  line L564 (-22.068, 33.313) -> (-22.068, 33.188)
  line L565 (-23.285, 36.643) -> (-24.627, 34.356)
  line L566 (-24.627, 34.356) -> (-24.975, 33.834)
  line L567 (-24.975, 33.834) -> (-25.025, 33.834)
  line L568 (-25.025, 33.834) -> (-25.099, 33.909)
  line L569 (-25.099, 33.909) -> (-26.715, 36.643)
  line L570 (-26.715, 36.643) -> (-26.715, 36.767)
  line L571 (-26.715, 36.767) -> (-26.541, 37.289)
  line L572 (-26.541, 37.289) -> (-26.441, 37.488)
  line L573 (-26.441, 37.488) -> (-26.367, 37.786)
  line L574 (-26.367, 37.786) -> (-26.118, 38.407)
  line L575 (-26.118, 38.407) -> (-26.093, 38.556)
  line L576 (-26.093, 38.556) -> (-25.025, 41.563)
  line L577 (-25.025, 41.563) -> (-24.95, 41.538)
  line L578 (-24.95, 41.538) -> (-24.553, 40.345)
  line L579 (-24.553, 40.345) -> (-24.428, 40.072)
  line L580 (-24.428, 40.072) -> (-24.031, 38.854)
  line L581 (-24.031, 38.854) -> (-23.285, 36.792)
  line L582 (-23.285, 36.792) -> (-23.285, 36.643)
  line L583 (-17.396, 16.588) -> (-17.42, 16.513)
  line L584 (-17.42, 16.513) -> (-18.315, 16.513)
  line L585 (-18.315, 16.513) -> (-19.11, 17.756)
  line L586 (-19.11, 17.756) -> (-20.005, 19.471)
  line L587 (-20.005, 19.471) -> (-20.775, 21.384)
  line L588 (-20.775, 21.384) -> (-21.049, 22.204)
  line L589 (-21.049, 22.204) -> (-21.372, 23.397)
  line L590 (-21.372, 23.397) -> (-21.695, 25.087)
  line L591 (-21.695, 25.087) -> (-21.869, 26.876)
  line L592 (-21.869, 26.876) -> (-21.894, 28.367)
  line L593 (-21.894, 28.367) -> (-21.745, 30.306)
  line L594 (-21.745, 30.306) -> (-21.521, 31.648)
  line L595 (-21.521, 31.648) -> (-21.248, 32.89)
  line L596 (-21.248, 32.89) -> (-20.85, 34.307)
  line L597 (-20.85, 34.307) -> (-20.403, 35.649)
  line L598 (-20.403, 35.649) -> (-19.756, 37.363)
  line L599 (-19.756, 37.363) -> (-18.738, 39.824)
  line L600 (-18.738, 39.824) -> (-16.923, 43.651)
  line L601 (-16.923, 43.651) -> (-16.849, 43.725)
  line L602 (-16.849, 43.725) -> (-14.513, 43.725)
  line L603 (-14.513, 43.725) -> (-14.389, 43.675)
  line L604 (-14.389, 43.675) -> (-14.438, 43.551)
  line L605 (-14.438, 43.551) -> (-15.134, 42.706)
  line L606 (-15.134, 42.706) -> (-16.302, 41.141)
  line L607 (-16.302, 41.141) -> (-17.744, 39.003)
  line L608 (-17.744, 39.003) -> (-18.564, 37.587)
  line L609 (-18.564, 37.587) -> (-19.036, 36.667)
  line L610 (-19.036, 36.667) -> (-19.756, 35.027)
  line L611 (-19.756, 35.027) -> (-20.303, 33.462)
  line L612 (-20.303, 33.462) -> (-20.75, 31.697)
  line L613 (-20.75, 31.697) -> (-20.974, 30.43)
  line L614 (-20.974, 30.43) -> (-21.123, 28.79)
  line L615 (-21.123, 28.79) -> (-21.123, 27.15)
  line L616 (-21.123, 27.15) -> (-21.049, 26.081)
  line L617 (-21.049, 26.081) -> (-20.85, 24.665)
  line L618 (-20.85, 24.665) -> (-20.676, 23.844)
  line L619 (-20.676, 23.844) -> (-20.328, 22.527)
  line L620 (-20.328, 22.527) -> (-20.055, 21.682)
  line L621 (-20.055, 21.682) -> (-19.657, 20.639)
  line L622 (-19.657, 20.639) -> (-19.235, 19.669)
  line L623 (-19.235, 19.669) -> (-18.713, 18.626)
  line L624 (-18.713, 18.626) -> (-18.067, 17.532)
  line L625 (-18.067, 17.532) -> (-17.396, 16.588)
  line L626 (-27.46, 20.365) -> (-27.038, 20.937)
  line L627 (-27.038, 20.937) -> (-26.938, 20.987)
  line L628 (-26.938, 20.987) -> (-25.422, 17.855)
  line L629 (-25.422, 17.855) -> (-25.447, 17.681)
  line L630 (-25.447, 17.681) -> (-25.646, 17.309)
  line L631 (-25.646, 17.309) -> (-26.168, 16.513)
  line L632 (-26.168, 16.513) -> (-30.716, 16.513)
  line L633 (-30.716, 16.513) -> (-30.741, 16.588)
  line L634 (-30.741, 16.588) -> (-29.001, 18.526)
  line L635 (-29.001, 18.526) -> (-27.46, 20.365)
  line L636 (-27.485, 36.692) -> (-27.485, 36.568)
  line L637 (-27.485, 36.568) -> (-28.33, 34.158)
  line L638 (-28.33, 34.158) -> (-28.429, 34.207)
  line L639 (-28.429, 34.207) -> (-28.926, 35.798)
  line L640 (-28.926, 35.798) -> (-29.771, 38.059)
  line L641 (-29.771, 38.059) -> (-31.064, 41.166)
  line L642 (-31.064, 41.166) -> (-32.182, 43.601)
  line L643 (-32.182, 43.601) -> (-32.182, 43.675)
  line L644 (-32.182, 43.675) -> (-32.132, 43.725)
  line L645 (-32.132, 43.725) -> (-31.287, 43.725)
  line L646 (-31.287, 43.725) -> (-31.138, 43.675)
  line L647 (-31.138, 43.675) -> (-30.517, 42.259)
  line L648 (-30.517, 42.259) -> (-29.672, 40.569)
  line L649 (-29.672, 40.569) -> (-28.131, 37.786)
  line L650 (-28.131, 37.786) -> (-27.485, 36.692)
  line L651 (-13.4958, 46.0631) -> (-12.202, 45.291)
  line L652 (-12.202, 45.291) -> (-11.034, 44.496)
  line L653 (-11.034, 44.496) -> (-11.009, 44.421)
  line L654 (-11.009, 44.421) -> (-19.21, 44.396)
  line L655 (-19.21, 44.396) -> (-19.284, 44.322)
  line L656 (-19.284, 44.322) -> (-19.856, 42.806)
  line L657 (-19.856, 42.806) -> (-20.577, 41.339)
  line L658 (-20.577, 41.339) -> (-22.44, 38.059)
  line L659 (-22.44, 38.059) -> (-22.763, 37.562)
  line L660 (-22.763, 37.562) -> (-22.763, 37.512)
  line L661 (-22.763, 37.512) -> (-22.838, 37.488)
  line L662 (-22.838, 37.488) -> (-23.285, 38.68)
  line L663 (-23.285, 38.68) -> (-23.36, 38.979)
  line L664 (-23.36, 38.979) -> (-24.627, 42.582)
  line L665 (-24.627, 42.582) -> (-24.578, 42.88)
  line L666 (-24.578, 42.88) -> (-24.453, 43.154)
  line L667 (-24.453, 43.154) -> (-24.105, 44.222)
  line L668 (-24.105, 44.222) -> (-24.105, 44.322)
  line L669 (-24.105, 44.322) -> (-24.18, 44.396)
  line L670 (-24.18, 44.396) -> (-25.82, 44.396)
  line L671 (-25.82, 44.396) -> (-25.895, 44.322)
  line L672 (-25.895, 44.322) -> (-25.895, 44.197)
  line L673 (-25.895, 44.197) -> (-25.373, 42.731)
  line L674 (-25.373, 42.731) -> (-25.373, 42.557)
  line L675 (-25.373, 42.557) -> (-26.044, 40.619)
  line L676 (-26.044, 40.619) -> (-26.143, 40.42)
  line L677 (-26.143, 40.42) -> (-26.466, 39.376)
  line L678 (-26.466, 39.376) -> (-26.864, 38.333)
  line L679 (-26.864, 38.333) -> (-27.112, 37.537)
  line L680 (-27.112, 37.537) -> (-27.187, 37.512)
  line L681 (-27.187, 37.512) -> (-27.584, 38.159)
  line L682 (-27.584, 38.159) -> (-29.125, 40.942)
  line L683 (-29.125, 40.942) -> (-29.896, 42.532)
  line L684 (-29.896, 42.532) -> (-30.542, 44.098)
  line L685 (-30.542, 44.098) -> (-30.591, 44.297)
  line L686 (-30.591, 44.297) -> (-30.691, 44.396)
  line L687 (-39.041, 44.396) -> (-39.0593, 44.4509)
  arc A8 (-14.7269, 46.6902) -> (-39.0593, 44.4509) centre (-25, 25) ccw
  line L688 (-14.7269, 46.6902) -> (-13.8205, 46.2372)
  arc A9 (-13.4958, 46.0631) -> (-13.8205, 46.2372) centre (-25, 25) ccw
  line L689 (-13.345, 43.725) -> (-12.202, 43.7)
  line L690 (-12.202, 43.7) -> (-12.177, 43.626)
  line L691 (-12.177, 43.626) -> (-12.873, 42.831)
  line L692 (-12.873, 42.831) -> (-14.041, 41.389)
  line L693 (-14.041, 41.389) -> (-15.209, 39.824)
  line L694 (-15.209, 39.824) -> (-16.725, 37.587)
  line L695 (-16.725, 37.587) -> (-17.57, 36.17)
  line L696 (-17.57, 36.17) -> (-18.265, 34.829)
  line L697 (-18.265, 34.829) -> (-18.912, 33.263)
  line L698 (-18.912, 33.263) -> (-19.284, 32.045)
  line L699 (-19.284, 32.045) -> (-19.607, 30.504)
  line L700 (-19.607, 30.504) -> (-19.756, 28.939)
  line L701 (-19.756, 28.939) -> (-19.732, 26.976)
  line L702 (-19.732, 26.976) -> (-19.657, 26.205)
  line L703 (-19.657, 26.205) -> (-19.483, 25.112)
  line L704 (-19.483, 25.112) -> (-19.011, 23.223)
  line L705 (-19.011, 23.223) -> (-18.588, 22.03)
  line L706 (-18.588, 22.03) -> (-18.265, 21.26)
  line L707 (-18.265, 21.26) -> (-17.42, 19.57)
  line L708 (-17.42, 19.57) -> (-17.048, 18.949)
  line L709 (-17.048, 18.949) -> (-16.327, 17.93)
  line L710 (-16.327, 17.93) -> (-15.755, 17.234)
  line L711 (-15.755, 17.234) -> (-15.184, 16.663)
  line L712 (-15.184, 16.663) -> (-15.209, 16.563)
  line L713 (-15.209, 16.563) -> (-16.377, 16.513)
  line L714 (-16.377, 16.513) -> (-16.998, 17.259)
  line L715 (-16.998, 17.259) -> (-17.445, 17.905)
  line L716 (-17.445, 17.905) -> (-18.34, 19.471)
  line L717 (-18.34, 19.471) -> (-18.738, 20.316)
  line L718 (-18.738, 20.316) -> (-19.433, 22.105)
  line L719 (-19.433, 22.105) -> (-19.781, 23.248)
  line L720 (-19.781, 23.248) -> (-20.055, 24.366)
  line L721 (-20.055, 24.366) -> (-20.204, 25.186)
  line L722 (-20.204, 25.186) -> (-20.353, 26.379)
  line L723 (-20.353, 26.379) -> (-20.403, 27.1)
  line L724 (-20.403, 27.1) -> (-20.403, 28.914)
  line L725 (-20.403, 28.914) -> (-20.204, 30.728)
  line L726 (-20.204, 30.728) -> (-20.005, 31.747)
  line L727 (-20.005, 31.747) -> (-19.682, 33.014)
  line L728 (-19.682, 33.014) -> (-19.11, 34.704)
  line L729 (-19.11, 34.704) -> (-18.415, 36.295)
  line L730 (-18.415, 36.295) -> (-18.091, 36.941)
  line L731 (-18.091, 36.941) -> (-17.371, 38.208)
  line L732 (-17.371, 38.208) -> (-15.855, 40.519)
  line L733 (-15.855, 40.519) -> (-14.861, 41.861)
  line L734 (-14.861, 41.861) -> (-13.419, 43.675)
  line L735 (-13.419, 43.675) -> (-13.345, 43.725)
  arc A10 (-41.6193, 7.6853) -> (-25.5, 1.0052) centre (-25, 25) ccw
  line L736 (-41.6193, 7.6853) -> (-42.3147, 8.3807)
  arc A11 (-46.9999, 15.4081) -> (-42.3147, 8.3807) centre (-25, 25) ccw
  line L737 (-38.8766, 43.7125) -> (-37.798, 42.458)
  line L738 (-37.798, 42.458) -> (-36.481, 40.842)
  line L739 (-36.481, 40.842) -> (-35.065, 38.904)
  line L740 (-35.065, 38.904) -> (-33.847, 37.09)
  line L741 (-33.847, 37.09) -> (-33.151, 35.922)
  line L742 (-33.151, 35.922) -> (-32.43, 34.53)
  line L743 (-32.43, 34.53) -> (-31.884, 33.213)
  line L744 (-31.884, 33.213) -> (-31.486, 31.971)
  line L745 (-31.486, 31.971) -> (-31.238, 30.902)
  line L746 (-31.238, 30.902) -> (-31.088, 29.908)
  line L747 (-31.088, 29.908) -> (-30.989, 28.442)
  line L748 (-30.989, 28.442) -> (-31.039, 26.951)
  line L749 (-31.039, 26.951) -> (-31.163, 25.932)
  line L750 (-31.163, 25.932) -> (-31.486, 24.317)
  line L751 (-31.486, 24.317) -> (-31.884, 22.975)
  line L752 (-31.884, 22.975) -> (-32.306, 21.856)
  line L753 (-32.306, 21.856) -> (-32.878, 20.614)
  line L754 (-32.878, 20.614) -> (-33.524, 19.471)
  line L755 (-33.524, 19.471) -> (-34.418, 18.203)
  line L756 (-34.418, 18.203) -> (-34.866, 17.681)
  line L757 (-34.866, 17.681) -> (-35.661, 16.911)
  line L758 (-35.661, 16.911) -> (-35.835, 16.936)
  line L759 (-35.835, 16.936) -> (-36.332, 17.259)
  line L760 (-36.332, 17.259) -> (-37.028, 17.955)
  line L761 (-37.028, 17.955) -> (-37.525, 18.725)
  line L762 (-37.525, 18.725) -> (-37.724, 19.123)
  line L763 (-37.724, 19.123) -> (-38.047, 19.943)
  line L764 (-38.047, 19.943) -> (-38.37, 21.185)
  line L765 (-38.37, 21.185) -> (-38.494, 21.956)
  line L766 (-38.494, 21.956) -> (-38.593, 23.149)
  line L767 (-38.593, 23.149) -> (-38.593, 26.628)
  line L768 (-38.593, 26.628) -> (-38.544, 26.677)
  line L769 (-38.544, 26.677) -> (-38.419, 26.702)
  line L770 (-38.419, 26.702) -> (-38.345, 26.827)
  line L771 (-38.345, 26.827) -> (-38.345, 33.014)
  line L772 (-38.345, 33.014) -> (-38.469, 33.139)
  line L773 (-38.469, 33.139) -> (-39.438, 33.114)
  line L774 (-39.438, 33.114) -> (-39.538, 32.99)
  line L775 (-39.538, 32.99) -> (-39.538, 26.851)
  line L776 (-39.538, 26.851) -> (-39.438, 26.702)
  line L777 (-39.438, 26.702) -> (-39.289, 26.628)
  line L778 (-39.289, 26.628) -> (-39.289, 22.975)
  line L779 (-39.289, 22.975) -> (-39.115, 21.334)
  line L780 (-39.115, 21.334) -> (-38.991, 20.688)
  line L781 (-38.991, 20.688) -> (-38.792, 19.943)
  line L782 (-38.792, 19.943) -> (-38.593, 19.346)
  line L783 (-38.593, 19.346) -> (-38.196, 18.452)
  line L784 (-38.196, 18.452) -> (-37.898, 17.93)
  line L785 (-37.898, 17.93) -> (-37.5, 17.383)
  line L786 (-37.5, 17.383) -> (-37.053, 16.911)
  line L787 (-37.053, 16.911) -> (-36.506, 16.513)
  line L788 (-36.506, 16.513) -> (-36.407, 16.414)
  line L789 (-36.407, 16.414) -> (-36.407, 16.364)
  line L790 (-36.407, 16.364) -> (-36.754, 16.116)
  line L791 (-36.754, 16.116) -> (-37.475, 15.743)
  line L792 (-37.475, 15.743) -> (-38.221, 15.47)
  line L793 (-38.221, 15.47) -> (-38.345, 15.47)
  line L794 (-38.345, 15.47) -> (-39.24, 15.867)
  line L795 (-39.24, 15.867) -> (-39.911, 16.29)
  line L796 (-39.911, 16.29) -> (-40.432, 16.712)
  line L797 (-40.432, 16.712) -> (-41.252, 17.582)
  line L798 (-41.252, 17.582) -> (-41.625, 18.104)
  line L799 (-41.625, 18.104) -> (-41.998, 18.75)
  line L800 (-41.998, 18.75) -> (-42.271, 19.322)